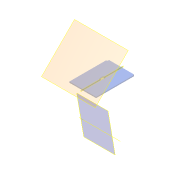
# Autodesk Inventor part: 00_Comar_Dichroic_16x25x0.2
Saved by Autodesk Inventor 2019.4 (Build 234330000, 330)
## iProperties
Created: 2019-08-10
Part Number: 00_Comar_Dichroic_16x25x0.2
Material: Glas
Document SubType Name: Modeling
Designer: diederichbenedict
Density: 2.18 g/cm^3
Appearance: Klar - Blau
Author: diederichbenedict
Autodesk Inventor part; units mm, degrees
ref_plane "YZ Plane" through (0, 0, 0) normal (1, 0, 0) x (0, 1, 0)
ref_plane "XZ Plane" through (0, 0, 0) normal (0, 1, 0) x (-1, 0, 0)
ref_plane "XY Plane" through (0, 0, 0) normal (0, 0, 1) x (1, 0, 0)
sketch "Sketch1" plane through (0, 0, 0) normal (0, 1, 0) x (-1, 0, 0)
  circle A0 centre (8, -12.5) radius 1.1261
  line L0 (-4.5, -30.5) -> (20.5, -30.5)
  line L1 (20.5, -30.5) -> (20.5, 5.5)
  line L2 (20.5, 5.5) -> (-4.5, 5.5)
  line L3 (-4.5, 5.5) -> (-4.5, -30.5)
  line L4 (-4.5, -30.5) -> (20.5, 5.5) construction
  line L5 (20.5, -30.5) -> (-4.5, 5.5) construction
  dimension "d7" = 25
  dimension "d8" = 36
  constraints: 12 end point, 2 midpoint, 2 parallel, 1 centre point, 1 horizontal, 1 perpendicular
  measures "d7" distance of L2.end L1.end
  measures "d8" distance of L1.end L0.end
extrude "Extrusion1" add sketch "Sketch1" along normal blind 1
ref_plane "Work Plane1" through (16.9, 36.305, -11.9513) normal (0, 0.7071, 0.7071) x (-1, 0, 0)
sketch "Sketch2" plane through (16.9, 36.305, -11.9513) normal (0, 0.7071, 0.7071) x (-1, 0, 0)
  ellipse E0 centre (24.9, 24.5764) end of major axis (23.7739, 24.5764) minor radius 0.7963 projected
  circle A0 centre (24.9, 24.9) radius 1.1798
  ellipse E1 centre (24.9, 25.2835) end of major axis (23.7739, 25.2835) minor radius 0.7963 projected
  line L0 (12.4, 11.8485) -> (37.4, 11.8485) projected
  circle A1 centre (37.4, 11.8485) radius 1.2055
  circle A2 centre (12.4, 11.8485) radius 0.8893
  point P0 (16.9, 34.1223)
  dimension "d4" = 0.3236
  constraints: 3 centre point, 1 coincident, 3 other
  measures "d4" distance of point (24.9, 24.576) A0.centre
extrude "Extrusion2" cut sketch "Sketch2" against normal through all contours E0 E1 A0 | E0 A0 E1 | E1 A0 E0 | E0 E1 | E0 A0 | E1 A0 E0 | A1 | A2 picked at (24.9476, 23.7672)
ref_plane "Work Plane2" through (-8, 0, -30.5) normal (-1, 0, 0) x (0, 0, 1)
ref_plane "Work Plane3" through (4, -7.358, 16.4985) normal (-0.7071, -0.5, 0.5) x (0.7071, -0.5, 0.5)
ref_plane "Work Plane4" through (4, -34.1432, -4.941) normal (0, -0.7071, 0.7071) x (1, 0, 0)
sketch "Sketch3" plane through (4, -34.1432, -4.941) normal (0, -0.7071, 0.7071) x (1, 0, 0)
  arc A0 (-13.1253, 18.7686) -> (-10.8747, 18.7686) centre (-12, 18.4144) ccw projected
  circle A1 centre (-12, 18.4144) radius 1.1798
  point P0 (-4, 27.6367)
  constraints: 1 centre point, 1 coincident, 1 concentric
extrude "Extrusion3" cut sketch "Sketch3" against normal through all
body "Solid1"
